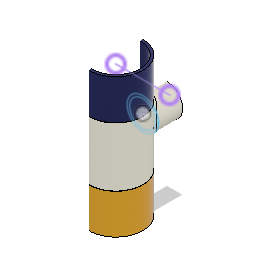
Two Way Valve (Autodesk Fusion 360 design; units mm, degrees)
Autodesk Fusion 360 part; units mm, degrees
sketch "Sketch1" plane through (0, 0, 0) normal (0, 1, 0) x (1, 0, 0)
  circle A0 centre (0, 0) radius 14
  circle A1 centre (0, 0) radius 15.5
  dimension "d1" = 28
  dimension "d2" = 1.5
  constraint coincident A0.centre A1.centre
  measures "d1" diameter of A0
  measures "d2" distance of A0 A1
extrude "Extrude1" add sketch "Sketch1" along normal blind 40 makes body 1
ref_plane "WorkPlane1" through (0, 21.655, -15.5) normal (0, 0, -1) x (1, 0, 0)
sketch "Sketch2" plane through (0, 21.655, -15.5) normal (0, 0, -1) x (1, 0, 0)
  circle A0 centre (0, -1.345) radius 7.5
  circle A1 centre (0, -1.345) radius 9
  line L0 (-15.5, -18.345) -> (15.5, -18.345)
  dimension "d6" = 15
  dimension "d7" = 1.5
  dimension "d14" = 17
  constraint concentric A0 A1
  measures "d6" diameter of A0
  measures "d7" distance of A0 A1
  measures "d14" distance of A0.centre L0
extrude "Extrude3" cut sketch "Sketch2" along normal mid plane 16 contours A0 bodies 1
extrude "Extrude2" add sketch "Sketch2" along normal blind 14 and the other way blind 5 bodies 1
copy_body "Body->Comp1" bodies 1 removing the originals makes body 2 in component "Valve"
fillet "Fillet1" radius 4 1 edges at (9, 23, -12.6194) on bodies 2 in component "Valve"
ref_plane "WorkPlane2" through (0, 13, 0) normal (0, -1, 0) x (-1, 0, 0)
sketch "Sketch3" plane through (0, 13, 0) normal (0, -1, 0) x (1, 0, 0)
  circle A0 centre (0, 0) radius 14
  circle A1 centre (0, 0) radius 14
  constraint coincident A0.centre A1.centre
  constraint equal A0 A1
extrude "Extrude4" add sketch "Sketch3" against normal blind 1.5 separate body makes body 3
copy_body "CutPasteBodies1" bodies 3 removing the originals makes body 4 in component "Valve"
ref_plane "WorkPlane3" through (0, 14.5, 0) normal (0, 1, 0) x (-1, 0, 0)
sketch "Sketch4" plane through (0, 14.5, 0) normal (0, 1, 0) x (1, 0, 0)
  circle A0 centre (0, 0) radius 7
  circle A1 centre (0, 0) radius 6
  dimension "d20" = 14
  dimension "d21" = 1
  constraint coincident A0.centre A1.centre
  constraint concentric A0 A1
  measures "d20" diameter of A0
  measures "d21" distance of A0 A1
extrude "Extrude1'" add sketch "Sketch4" along normal up to surface (20.5 mm away) bodies 4 in component "Valve"
extrude "Extrude2'" cut 1 faces at (0.9498, 14.5, 1.0623) along direction (0, -1, 0) blind 1.5 on bodies 4 bodies 4 in component "Valve"
fillet "Fillet2" radius 7 1 edges at (-6.5263, 14.5, -2.5313) on bodies 4 in component "Valve"
ref_plane "WorkPlane4" through (0, 13, 0) normal (0, -1, 0) x (1, 0, 0)
sketch "Sketch5" plane through (0, 13, 0) normal (0, -1, 0) x (1, 0, 0)
  circle A0 centre (0, 0) radius 11
  circle A1 centre (0, 0) radius 14
  circle A2 centre (0, 0) radius 6
  circle A3 centre (0, 0) radius 6
  circle A4 centre (0, 0) radius 10
  dimension "d28" = 3
  dimension "d29" = 1
  constraint coincident A0.centre A1.centre
  constraint concentric A0 A2
  constraint equal A2 A3
  constraint concentric A1 A4
  measures "d28" distance of A0 A1
  measures "d29" distance of A0 A4
extrude "Extrude3'" add sketch "Sketch5" along normal up to surface (9 mm away) contours A0 bodies 4 in component "Valve"
ref_plane "WorkPlane5" through (0, 13, 0) normal (0, -1, 0) x (1, 0, 0)
sketch "Sketch6" plane through (0, 13, 0) normal (0, -1, 0) x (1, 0, 0)
  line L0 (0, 0) -> (16.466, 0) construction
  line L1 (0, 0) -> (0, 11.3687) construction
  line L2 (10, 0.5) -> (3, 0.5)
  line L3 (3, 0.5) -> (3, -0.5)
  line L4 (3, -0.5) -> (10, -0.5)
  line L5 (10, -0.5) -> (10, 0.5)
  line L6 (10, 0.5) -> (3, -0.5) construction
  line L7 (3, 0.5) -> (10, -0.5) construction
  circle A0 centre (0, 0) radius 10
  line L8 (0.5, 10) -> (-0.5, 10)
  line L9 (-0.5, 10) -> (-0.5, 3)
  line L10 (-0.5, 3) -> (0.5, 3)
  line L11 (0.5, 3) -> (0.5, 10)
  line L12 (0.5, 10) -> (-0.5, 3) construction
  line L13 (-0.5, 10) -> (0.5, 3) construction
  line L14 (-0.5, -10) -> (0.5, -3) construction
  line L15 (0.5, -3) -> (0.5, -10)
  line L16 (0.5, -10) -> (-0.5, -3) construction
  line L17 (-0.5, -3) -> (0.5, -3)
  line L18 (0.5, -10) -> (-0.5, -10)
  line L19 (-0.5, -10) -> (-0.5, -3)
  line L20 (-10, -0.5) -> (-10, 0.5)
  line L21 (-3, 0.5) -> (-10, -0.5) construction
  line L22 (-10, 0.5) -> (-3, 0.5)
  line L23 (-3, -0.5) -> (-10, -0.5)
  line L24 (-3, 0.5) -> (-3, -0.5)
  line L25 (-10, 0.5) -> (-3, -0.5) construction
  point P0 (6.5, 0)
  point P1 (0, 6.5)
  point P2 (0, -6.5)
  point P3 (-6.5, 0)
  dimension "d33" = 7
  dimension "d34" = 1
  constraint coincident L0.start L1.start
  constraint horizontal L0
  constraint perpendicular L0 L1
  constraint horizontal L2
  constraint perpendicular L2 L3
  constraint parallel L2 L4
  constraint parallel L3 L5
  constraint coincident L6 P0
  constraint coincident L7 P0
  constraint coincident L0 P0
  constraint tangent L5 A0
  constraint horizontal L8
  constraint perpendicular L8 L9
  constraint parallel L8 L10
  constraint parallel L9 L11
  constraint coincident L12 P1
  constraint coincident L13 P1
  constraint coincident L1 P1
  constraint tangent A0 L8
  constraint equal L3 L10
  constraint equal L2 L11
  constraint symmetric L0 L8.start L15.end
  constraint symmetric L0 L8.end L14.start
  constraint symmetric L0 L9.end L16.end
  constraint symmetric L0 L10.end L14.end
  constraint symmetric L0 P1 P2
  constraint symmetric L1 L2.start L20.end
  constraint symmetric L1 L2.end L21.start
  constraint symmetric L1 L3.end L23.start
  constraint symmetric L1 L4.end L20.start
  constraint symmetric L1 P0 P3
  measures "d33" distance of L2.start L2.end
  measures "d34" distance of L2.end L3.end
extrude "Extrude4'" add sketch "Sketch6" along normal up to surface (9 mm away) contours L2 L3 L4 A0 | A0 L9 L10 L11 | A0 L15 L17 L19 | A0 L22 L23 L24 bodies 4 in component "Valve"
ref_plane "WorkPlane6" through (0, 4, 0) normal (0, -1, 0) x (0, 0, -1)
sketch "Sketch7" plane through (0, 4, 0) normal (0, -1, 0) x (1, 0, 0)
  circle A0 centre (0, 0) radius 1.25
  circle A1 centre (0, 0) radius 3.0414
  point P0 (-0.5, 3)
  dimension "d46" = 2.5
  constraint coincident A0.centre A1.centre
  constraint concentric A0 A1
  constraint coincident A1 P0
  measures "d46" diameter of A0
extrude "Extrude5" add sketch "Sketch7" against normal blind 3 bodies 4 in component "Valve"
fillet "Fillet3" radius 2 4 edges at (0, 7, 3) (-3, 7, 0) (0, 7, -3) (3, 7, 0) on bodies 4 in component "Valve"
fillet "Fillet5" radius 4 4 edges at (7.0711, 13, -7.0711) (-7.0711, 13, -7.0711) (7.0711, 13, 7.0711) (-7.0711, 13, 7.0711) on bodies 4 in component "Valve"
chamfer "Chamfer1" distance 2.5 angle 45 4 edges at (0, 13, 3) (3, 13, 0) (-3, 13, 0) (0, 13, -3) on bodies 4 in component "Valve"
fillet "Fillet6" radius 2 1 edges at (-8.3909, 19.7455, -10.5) on bodies 2 in component "Valve"
fillet "Fillet7" radius 2 5 edges at (0, 32, -14) (0, 14, -14) (-8.5056, 22.9981, -11.12) (0, 32, -14) (8.5056, 23.0019, -11.12) on bodies 2 in component "Valve"
ref_plane "WorkPlane7" through (0, 3.9, 0) normal (0, -1, 0) x (0, 0, -1)
sketch "Sketch8" plane through (0, 3.9, 0) normal (0, -1, 0) x (1, 0, 0)
  circle A0 centre (0, 0) radius 1.15
  circle A1 centre (0, 0) radius 1.25
  dimension "d48" = 0.1
  constraint coincident A0.centre A1.centre
  measures "d48" distance of A0 A1
extrude "Extrude5'" add sketch "Sketch8" against normal blind 3.25 separate body contours A0 makes body 5
copy_body "Body->Comp2" bodies 5 removing the originals makes body 6 in component "One-Way Gate Top"
ref_plane "WorkPlane8" through (0, 7.15, 0) normal (0, 1, 0) x (-1, 0, 0)
sketch "Sketch9" plane through (0, 7.15, 0) normal (0, 1, 0) x (1, 0, 0)
  circle A0 centre (0, 0) radius 1.24
  arc A1 (0.5, -1.1456) -> (1.1456, -0.5) centre (0, 0) ccw
  dimension "d52" = 0.01
  constraint coincident A0.centre A1.centre
  measures "d52" distance of A0 A1
ref_plane "WorkPlane9" through (0, 11.15, 0) normal (0, 1, 0) x (1, 0, 0)
sketch "Sketch10" plane through (0, 11.15, 0) normal (0, 1, 0) x (1, 0, 0)
  circle A0 centre (0, 0) radius 0.4
  dimension "d54" = 0.8
  constraint coincident A0.centre origin
  measures "d54" diameter of A0
loft "Loft1" add profiles "Sketch9", "Sketch10" section 1 section 2 bodies 6 in component "One-Way Gate Top"
fillet "Fillet1'" radius 0.25 1 edges at (-0.3729, 11.15, -0.1446) on bodies 6 in component "One-Way Gate Top"
ref_plane "WorkPlane10" through (0, 3.9, 0) normal (0, -1, 0) x (1, 0, 0)
sketch "Sketch11" plane through (0, 3.9, 0) normal (0, -1, 0) x (1, 0, 0)
  circle A0 centre (0, 0) radius 12.5
  arc A1 (5.9791, 0.5) -> (0.5, 5.9791) centre (0, 0) ccw
  circle A2 centre (0, 0) radius 11
  dimension "d60" = 1.5
  constraint coincident A0.centre A1.centre
  measures "d60" distance of A0 A2
extrude "Extrude1''" add sketch "Sketch11" along normal blind 0.05 contours A0 | A2 bodies 6 in component "One-Way Gate Top"
ref_plane "WorkPlane11" through (0, 0, 0) normal (0, -1, 0) x (-1, 0, 0)
sketch "Sketch12" plane through (0, 0, 0) normal (0, -1, 0) x (1, 0, 0)
  circle A0 centre (0, 0) radius 14.75
  circle A1 centre (0, 0) radius 15.5
  circle A2 centre (0, 0) radius 15.5
  line L0 (-15.5, 0) -> (-14, 0) construction
  circle A3 centre (0, 0) radius 14 construction
  line L1 (0, 0) -> (-5.9866, 0) construction
  point P0 (-14.75, 0)
  constraint coincident A0.centre A1.centre
  constraint equal A1 A2
  constraint horizontal L0
  constraint coincident A1 L0.start
  constraint coincident L0.end A3
  constraint horizontal L1
  constraint collinear L0 L1
  constraint coincident A0 P0
  constraint midpoint L0 P0
extrude "Extrude6" cut sketch "Sketch12" against normal blind 3 bodies 2 in component "Valve"
ref_plane "WorkPlane12" through (0, 2.9, 0) normal (0, -1, 0) x (1, 0, 0)
sketch "Sketch13" plane through (0, 2.9, 0) normal (0, -1, 0) x (1, 0, 0)
  circle A0 centre (0, 0) radius 15.5
  circle A1 centre (0, 0) radius 14.85
  circle A2 centre (0, 0) radius 14.75
  circle A3 centre (0, 0) radius 15.5
  dimension "d65" = 0.1
  constraint coincident A0.centre A1.centre
  constraint concentric A0 A1
  constraint equal A0 A3
  measures "d65" distance of A1 A2
extrude "Extrude6'" add sketch "Sketch13" along normal up to surface (2.9 mm away) separate body contours A0 A3 makes body 7
ref_plane "WorkPlane13" through (0, 0, 0) normal (0, -1, 0) x (0, 0, -1)
sketch "Sketch14" plane through (0, 0, 0) normal (0, -1, 0) x (1, 0, 0)
  circle A0 centre (0, 0) radius 15.5
  circle A1 centre (0, 0) radius 15.5
  circle A2 centre (0, 0) radius 14
  circle A3 centre (0, 0) radius 14
  constraint coincident A0.centre A1.centre
  constraint equal A0 A1
  constraint equal A2 A3
extrude "Extrude7" add sketch "Sketch14" along normal blind 20 bodies 7
copy_body "Body->Comp3" bodies 7 removing the originals makes body 8 in component "Tube Fit Top"
ref_plane "WorkPlane14" through (0, -3, 0) normal (0, -1, 0) x (-1, 0, 0)
sketch "Sketch15" plane through (0, -3, 0) normal (0, -1, 0) x (1, 0, 0)
  line L0 (1, 13.9642) -> (-1, 13.9642)
  line L1 (-1, 13.9642) -> (-1, -13.9642)
  line L2 (-1, -13.9642) -> (1, -13.9642)
  line L3 (1, -13.9642) -> (1, 13.9642)
  line L4 (1, 13.9642) -> (-1, -13.9642) construction
  line L5 (-1, 13.9642) -> (1, -13.9642) construction
  line L6 (13.9642, 1) -> (-13.9642, 1)
  line L7 (-13.9642, 1) -> (-13.9642, -1)
  line L8 (-13.9642, -1) -> (13.9642, -1)
  line L9 (13.9642, -1) -> (13.9642, 1)
  line L10 (13.9642, 1) -> (-13.9642, -1) construction
  line L11 (-13.9642, 1) -> (13.9642, -1) construction
  circle A0 centre (0, 0) radius 14
  circle A1 centre (0, 0) radius 2.5
  dimension "d72" = 2
  dimension "d75" = 5
  constraint horizontal L0
  constraint perpendicular L0 L1
  constraint parallel L0 L2
  constraint parallel L1 L3
  constraint coincident L4 A0.centre
  constraint coincident L5 A0.centre
  constraint coincident A0.centre A1.centre
  constraint horizontal L6
  constraint perpendicular L6 L7
  constraint parallel L6 L8
  constraint parallel L7 L9
  constraint coincident L10 A0.centre
  constraint coincident L11 A0.centre
  constraint equal L0 L9
  constraint coincident L0.start A0
  constraint coincident L6.start A0
  measures "d72" distance of L0.start L0.end
  measures "d75" diameter of A1
extrude "Extrude8" add sketch "Sketch15" along normal blind 3 separate body contours L0 L1 L3 A1 | L3 L6 A1 | L1 L3 L6 A1 | L6 L8 L9 A1 | L1 L6 A1 | L6 L7 L8 A1 | L3 L6 L8 A1 | L1 L3 L6 L8 | L1 L6 L8 A1 | L3 L8 A1 | L1 L3 L8 A1 | L1 L2 L3 A1 | L1 L8 A1 makes body 9
copy_body "CutPasteBodies1'" bodies 9 removing the originals makes body 10 in component "Tube Fit Top"
ref_plane "WorkPlane15" through (0, 40, 0) normal (0, 1, 0) x (1, 0, 0)
sketch "Sketch16" plane through (0, 40, 0) normal (0, 1, 0) x (1, 0, 0)
  circle A0 centre (0, 0) radius 14.75
  circle A1 centre (0, 0) radius 15.5
  circle A2 centre (0, 0) radius 15.5
  line L0 (0, 0) -> (-9.1726, 0) construction
  line L1 (-14, 0) -> (-15.5, 0) construction
  circle A3 centre (0, 0) radius 14 construction
  point P0 (-14.75, 0)
  constraint coincident A0.centre A1.centre
  constraint equal A1 A2
  constraint horizontal L0
  constraint horizontal L1
  constraint coincident A1 L1.end
  constraint coincident L1.start A3
  constraint collinear L0 L1
  constraint coincident A0 P0
  constraint midpoint L1 P0
extrude "Extrude7'" cut sketch "Sketch16" against normal blind 3 bodies 2 in component "Valve"
ref_plane "WorkPlane16" through (0, 37.1, 0) normal (0, 1, 0) x (1, 0, 0)
sketch "Sketch17" plane through (0, 37.1, -0.2552) normal (0, 1, 0) x (1, 0, 0)
  circle A0 centre (0, -0.2552) radius 7 construction
  circle A1 centre (0, -0.2552) radius 7 construction
  circle A2 centre (0, -0.2552) radius 14.85
  circle A3 centre (0, -0.2552) radius 15.5
  circle A4 centre (0, -0.2552) radius 14.75
  circle A5 centre (0, -0.2552) radius 15.5
  dimension "d80" = 0.1
  constraint equal A0 A1
  constraint tangent A0 A1
  constraint concentric A1 A2
  constraint concentric A2 A3
  constraint equal A3 A5
  measures "d80" distance of A2 A4
extrude "Extrude1'''" add sketch "Sketch17" along normal up to surface (3 mm away) separate body contours A3 A5 makes body 11 in component "Tube Fit Bottom"
ref_plane "WorkPlane17" through (0, 40.1, 0) normal (0, 1, 0) x (0, 0, 1)
sketch "Sketch18" plane through (0, 40.1, 0) normal (0, 1, 0) x (1, 0, 0)
  circle A0 centre (0, 0) radius 14
  circle A1 centre (0, 0) radius 15.5
  circle A2 centre (0, 0) radius 14
  circle A3 centre (0, 0) radius 15.5
  constraint coincident A0.centre A1.centre
  constraint concentric A0 A1
  constraint equal A0 A2
  constraint equal A1 A3
extrude "Extrude2''" add sketch "Sketch18" along normal blind 20 bodies 11 in component "Tube Fit Bottom"
ref_plane "WorkPlane18" through (0, 40.1, 0) normal (0, -1, 0) x (-1, 0, 0)
sketch "Sketch19" plane through (0, 40.1, 0) normal (0, -1, 0) x (1, 0, 0)
  circle A0 centre (0, 0) radius 5
  circle A1 centre (0, 0) radius 3.5
  dimension "d88" = 10
  dimension "d89" = 1.5
  constraint coincident A0.centre A1.centre
  measures "d88" diameter of A0
  measures "d89" distance of A0 A1
extrude "Extrude9" add sketch "Sketch19" against normal blind 3 separate body makes body 12
copy_body "CutPasteBodies1''" bodies 12 removing the originals makes body 13 in component "Tube Fit Bottom"
ref_plane "WorkPlane19" through (0, 43.1, 0) normal (0, 1, 0) x (-1, 0, 0)
sketch "Sketch20" plane through (0, 43.1, 0) normal (0, 1, 0) x (1, 0, 0)
  circle A0 centre (0, 0) radius 3.5
  circle A1 centre (0, 0) radius 5
  circle A2 centre (0, 0) radius 12.5
  circle A3 centre (0, 0) radius 14
  circle A4 centre (0, 0) radius 14
  circle A5 centre (0, 0) radius 3.5
  circle A6 centre (0, 0) radius 5
  line L0 (0, 0) -> (-20.1977, 0) construction
  line L1 (0, 0) -> (0, 16.0969) construction
  line L2 (-4.9434, 0.75) -> (-12.4775, 0.75)
  line L3 (-12.4775, -0.75) -> (-4.9434, -0.75)
  line L4 (-4.9434, 0.75) -> (-12.5, -0.75) construction
  line L5 (-12.5, 0.75) -> (-4.9434, -0.75) construction
  line L6 (-0.75, 12.4775) -> (-0.75, 4.9434)
  line L7 (0.75, 4.9434) -> (0.75, 12.4775)
  line L8 (0.75, 12.5) -> (-0.75, 4.9434) construction
  line L9 (-0.75, 12.5) -> (0.75, 4.9434) construction
  line L10 (0, 0) -> (0, -18.7282) construction
  line L11 (0, 0) -> (18.439, 0) construction
  line L12 (12.4775, 0.75) -> (4.9434, 0.75)
  line L13 (4.9434, -0.75) -> (12.4775, -0.75)
  line L14 (12.5, 0.75) -> (4.9434, -0.75) construction
  line L15 (4.9434, 0.75) -> (12.5, -0.75) construction
  line L16 (-0.75, -4.9434) -> (-0.75, -12.4775)
  line L17 (0.75, -12.4775) -> (0.75, -4.9434)
  line L18 (0.75, -4.9434) -> (-0.75, -12.5) construction
  line L19 (-0.75, -4.9434) -> (0.75, -12.5) construction
  point P0 (-8.7217, 0)
  point P1 (0, 8.7217)
  point P2 (8.7217, 0)
  point P3 (0, -8.7217)
  dimension "d93" = 1.5
  dimension "d94" = 1.5
  constraint coincident A0.centre A1.centre
  constraint concentric A1 A2
  constraint concentric A2 A3
  constraint equal A3 A4
  constraint equal A0 A5
  constraint equal A1 A6
  constraint horizontal L0
  constraint perpendicular L0 L1
  constraint horizontal L2
  constraint parallel L2 L3
  constraint coincident L4 P0
  constraint coincident L5 P0
  constraint coincident L0 P0
  constraint parallel L6 L7
  constraint coincident L8 P1
  constraint coincident L9 P1
  constraint coincident L1 P1
  constraint perpendicular L0 L10
  constraint perpendicular L10 L11
  constraint horizontal L12
  constraint parallel L12 L13
  constraint coincident L14 P2
  constraint coincident L15 P2
  constraint coincident L11 P2
  constraint parallel L16 L17
  constraint coincident L18 P3
  constraint coincident L19 P3
  constraint coincident L10 P3
  constraint coincident A1 L7.start
  constraint coincident A1 L12.end
  constraint coincident A1 L2.start
  constraint coincident A1 L16.start
  constraint coincident A2 L3.start
  constraint coincident A2 L2.end
  constraint coincident A2 L16.end
  constraint coincident A2 L17.start
  constraint coincident A2 L12.start
  constraint coincident A2 L13.end
  constraint coincident A2 L6.start
  constraint coincident A2 L7.end
  measures "d93" distance of A2 A3
  measures "d94" distance of L5.start L4.end
extrude "Extrude10" add sketch "Sketch20" along normal blind 1.5 separate body contours A1 A6 | A1 A2 A6 L12 L13 | A1 A2 A6 L6 L7 | A1 A2 A6 L16 L17 | A1 A2 A6 L2 L3 | A3 A4 makes body 14
copy_body "CutPasteBodies2" bodies 14 removing the originals makes body 15 in component "Tube Fit Bottom"
fillet "Fillet1''" radius 1 1 edges at (-3.2631, 40.1, 1.2657) on bodies 13 in component "Tube Fit Bottom"
fillet "Fillet2'" radius 0.5 1 edges at (-4.6616, 40.1, -1.8081) on bodies 13 in component "Tube Fit Bottom"
component "Valve" placed x (1, 0, 0) y (0, 1, 0) z (0, 0, 1) at (0, 0, 0)
component "One-Way Gate Top" placed x (1, 0, 0) y (0, 1, 0) z (0, 0, 1) at (0, 0, 0)
component "Tube Fit Top" placed x (1, 0, 0) y (0, 1, 0) z (0, 0, 1) at (0, 0, 0)
component "Tube Fit Bottom" placed x (1, 0, 0) y (0, 1, 0) z (0, 0, 1) at (0, 0, 0)
